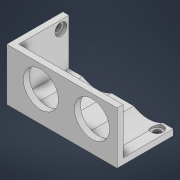
# Autodesk Inventor part: Buttons_Mount_v3
Saved by Autodesk Inventor 2022 (Build 260153000, 153)
## iProperties
Created: 2022-04-20
Part Number: Buttons_Mount_v3
Material: Generisch
Document SubType Name: Modeling
Designer: Martin
Density: 1 g/cm^3
Appearance: Vorgabe
Author: Martin
Autodesk Inventor part; units mm, degrees
ref_plane "YZ Plane" through (0, 0, 0) normal (1, 0, 0) x (0, 1, 0)
ref_plane "XZ Plane" through (0, 0, 0) normal (0, 1, 0) x (-1, 0, 0)
ref_plane "XY Plane" through (0, 0, 0) normal (0, 0, 1) x (1, 0, 0)
sketch "Skizze1" plane through (0, 0, 0) normal (0, 0, 1) x (1, 0, 0)
  line L0 (0, 0) -> (55, 0)
  line L1 (55, 0) -> (55, 26)
  line L2 (55, 26) -> (0, 26)
  line L3 (0, 26) -> (0, 0)
  circle A0 centre (17, 15) radius 8.75
  circle A1 centre (42.5, 15) radius 8.75
  dimension "D" = 17.5
  dimension "d1" = 17.5
  dimension "Hoehe" = 26
  dimension "L" = 55
  dimension "d5" = 17
  dimension "d7" = 11
  dimension "d14" = 12.5
  constraints: 8 end point, 2 centre point, 2 parallel, 1 horizontal, 1 horizontal alignment, 1 perpendicular
  measures "D" diameter of A0
  measures "d1" diameter of A1
  measures "Hoehe" distance of L0.end L1.end
  measures "L" distance of L1.end L2.end
  measures "d5" distance from line of L3 A0.centre
  measures "d7" distance from line of L2 A0.centre
  measures "d14" distance from line of L1 A1.centre
extrude "Extrusion1" add sketch "Skizze1" along normal blind 3
sketch "Skizze2" plane through (0, 0, 0) normal (0, 0, -1) x (-1, 0, 0)
  line L0 (-55, 0) -> (-55, 26) projected
  line L1 (0, 0) -> (-55, 0) projected
  line L2 (0, 26) -> (0, 0) projected
  line L3 (-55, 26) -> (0, 26) projected
  circle A0 centre (-17, 15) radius 8.75 projected
  circle A1 centre (-42.5, 15) radius 8.75 projected
  line L4 (-55, 26) -> (0, 26) projected
  line L5 (-3, 26) -> (-3, 3)
  line L6 (-3, 3) -> (-55, 3)
  dimension "Dicke" = 3
  dimension "d11" = 3
  constraints: 4 end point, 2 point on line, 1 perpendicular, 1 vertical
  measures "Dicke" distance between parallel lines of L2 L5
  measures "d11" distance between parallel lines of L1 L6
extrude "Extrusion2" add sketch "Skizze2" along normal blind 25 contours L0 L6 L5 L3 L2 L1
sketch "Skizze3" plane through (3, 3, 0) normal (0, 1, 0) x (1, 0, 0)
  line L0 (52, 0) -> (52, 25) projected
  line L1 (0, 25) -> (52, 25) projected
  point P0 (-3, 0)
  point P1 (48, 21)
  dimension "d22" = 4
  dimension "d23" = 4
  measures "d22" distance from line of L0 point (48, 21)
  measures "d23" distance from line of L1 point (48, 21)
hole "Bohrung1" at (51, 3, -21) direction (0, -1, 0) diameter 3.5 end through all counterbore diameter 6 counterbore depth 1.5
sketch "Skizze4" plane through (3, 3, 0) normal (1, 0, 0) x (0, 0, -1)
  line L0 (0, 23) -> (25, 23) projected
  line L1 (25, 23) -> (25, 0) projected
  point P0 (0, -3)
  point P1 (21, 19)
  dimension "d31" = 4
  dimension "d32" = 4
  measures "d31" distance from line of L0 point (21, 19)
  measures "d32" distance from line of L1 point (21, 19)
hole "Bohrung2" at (3, 22, -21) direction (-1, 0, 0) diameter 3.5 end through all counterbore diameter 6 counterbore depth 1.5
sketch "Skizze5" plane through (0, 0, -25) normal (0, 0, -1) x (-1, 0, 0)
  circle A0 centre (-42.5, 15) radius 8.75 projected
  circle A1 centre (-17, 15) radius 8.75 projected
  circle A2 centre (-42.5, 15) radius 14
  circle A3 centre (-17, 15) radius 14
  point P0 (0, 0)
  point P1 (-29.75, 9.2175)
  point P2 (-29.75, 20.7825)
  dimension "d33" = 28
  dimension "d34" = 28
  constraints: 2 centre point, 2 coincident
  measures "d33" diameter of A2
  measures "d34" diameter of A3
extrude "Extrusion3" cut sketch "Skizze5" against normal blind 25 contours A2 A3 | A3 A2 picked at (-4.9763, 13.1615) picked at (-54.5237, 16.8385)
equation "\"d1\" = D"
equation "\"d11\" = Dicke"
equation "\"d23\" = d22"
equation "\"d34\" = d33"
